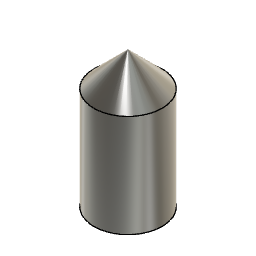
Cylindrical v4 (Autodesk Fusion 360 design; units mm, degrees)
Autodesk Fusion 360 part; units mm, degrees
cylinder "CylinderPrimitive1" add diameter 10 height 20 placed x (1, 0, 0) y (0, 1, 0) z (0, 0, 1) at (0, 0, 0)
chamfer "Chamfer1" distance 5 angle 45 1 edges at (-4.6616, -1.8081, 20)
component "Base" placed x (1, 0, 0) y (0, 1, 0) z (0, 0, 1) at (0, 0, 0)
